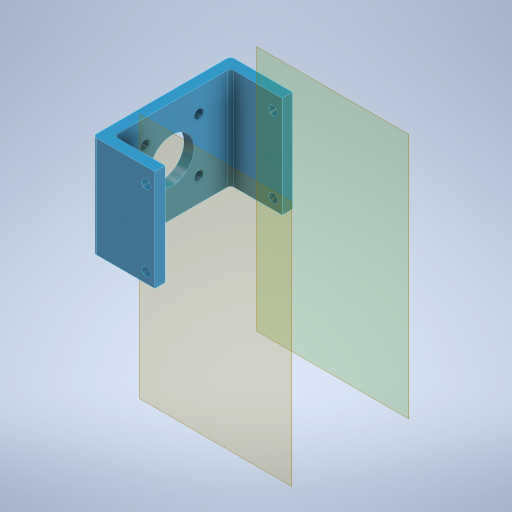
# Autodesk Inventor part: 3D_pelvis2
Saved by Autodesk Inventor 2024 (Build 280153000, 153)
## iProperties
Created: 2024-09-03
Part Number: 3D_pelvis2
Material: PMMA 플라스틱
Document SubType Name: Modeling
Designer: jmha0
Density: 1.188 g/cm^3
Appearance: 하늘색 짙음
Author: jmha0
Autodesk Inventor part; units mm, degrees
ref_plane "YZ Plane" through (0, 0, 0) normal (1, 0, 0) x (0, 1, 0)
ref_plane "XZ Plane" through (0, 0, 0) normal (0, 1, 0) x (-1, 0, 0)
ref_plane "XY Plane" through (0, 0, 0) normal (0, 0, 1) x (1, 0, 0)
ref_plane "작업 평면1" through (0, 0, -34) normal (0, 0, -1) x (-1, 0, 0)
sketch "스케치1" plane through (0, 0, -34) normal (0, 0, -1) x (-1, 0, 0)
  circle A0 centre (17.3, -18) radius 1.35 projected
  line L0 (20.1, -44.6) -> (20.1, 8.5) projected
  line L1 (14.5, -42) -> (14.5, 11.5) projected
  circle A1 centre (17.3, 4) radius 1.35 projected
  circle A2 centre (17.3, -18) radius 1.45
  circle A3 centre (17.3, 4) radius 1.45
  line L2 (14.7, -42) -> (14.7, 11.5)
  line L3 (14.7, 11.5) -> (20.1, 8.5)
  line L4 (14.7, -20.9546) -> (32.7, -20.9546)
  line L5 (32.7, -20.9546) -> (32.7, 8.5)
  line L6 (32.7, 8.5) -> (20.1, 8.5)
  line L7 (32.7, -20.9546) -> (26.7, -20.9546)
  line L8 (26.7, -20.9546) -> (26.7, 8.5)
  line L9 (26.7, 8.5) -> (32.7, 8.5)
  line L10 (32.7, 8.5) -> (32.7, -20.9546)
  line L11 (20.1, 8.5) -> (14.7, 8.5)
  point P0 (0, 0)
  dimension "d0" = 0.1
  dimension "d1" = 0.1
  dimension "d2" = 0.2
  dimension "d3" = 18
  dimension "d8" = 6
  constraints: 20 end point, 4 perpendicular, 4 point on line, 3 parallel, 2 centre point, 1 horizontal
  measures "d0" radial gap between concentric circles of A0 A2
  measures "d1" radial gap between concentric circles of A1 A3
  measures "d2" distance between parallel lines of L1 L2
  measures "d3" distance of L4.start L4.end
  measures "d8" distance of L8.end L9.end
extrude "돌출1" add sketch "스케치1" along normal blind 3 contours L4 L2 L11 L0 | L0 L6 L8 L4 | L8 L6 L5 L4 | A2 | A3
sketch "스케치2" plane through (0, 0, -34) normal (0, 0, 1) x (1, 0, 0)
  line L0 (-20.1, 8.5) -> (-14.7, 11.5) projected
  line L1 (-14.7, 8.5) -> (-14.7, -20.9546) projected
  line L2 (-20.1, -44.6) -> (-20.1, 8.5) projected
  line L3 (-32.7, 8.5) -> (-14.7, 8.5) projected
  line L4 (-32.7, -20.9546) -> (-32.7, 8.5) projected
  line L5 (-14.7, -20.9546) -> (-32.7, -20.9546) projected
  line L6 (-20.1, -20.9546) -> (-32.7, -20.9546)
  line L7 (-32.7, -20.9546) -> (-32.7, 8.5)
  line L8 (-32.7, 8.5) -> (-20.1, 8.5)
  line L9 (-20.1, 8.5) -> (-20.1, -20.9546)
  line L10 (-20.1, -20.9546) -> (-14.7, -20.9546)
  line L11 (-14.7, 11.5) -> (-20.1, 8.5)
  circle A0 centre (-17.3, -18) radius 1.45 projected
  circle A1 centre (-17.3, 4) radius 1.35 projected
  circle A2 centre (-17.3, 4) radius 1.45 projected
  circle A3 centre (-17.3, 4) radius 1.45
  circle A4 centre (-17.3, -18) radius 1.45
  point P0 (0, 0)
  constraints: 12 end point, 2 centre point, 2 coincident, 2 concentric, 2 parallel, 2 point on line, 1 collinear, 1 horizontal, 1 perpendicular
ref_plane "작업 평면2" through (0, 0, 0) normal (0, 0, 1) x (1, 0, 0)
sketch "스케치3" plane through (0, 0, 0) normal (0, 0, 1) x (1, 0, 0)
  line L0 (-32.7, 8.5) -> (-14.7, 8.5) projected
  line L1 (-32.7, -20.9546) -> (-32.7, 8.5) projected
  line L2 (-14.7, -20.9546) -> (-32.7, -20.9546) projected
  line L3 (-14.7, 8.5) -> (-14.7, -20.9546) projected
  line L4 (-20.1, -20.9546) -> (-32.7, -20.9546)
  line L5 (-32.7, -20.9546) -> (-32.7, 8.5)
  line L6 (-32.7, 8.5) -> (-20.1, 8.5)
  line L7 (-20.1, 8.5) -> (-20.1, -20.9546)
  line L8 (-32.7, -20.9546) -> (-20.1, -20.9546)
  line L9 (-20.1, -20.9546) -> (-20.1, 8.5)
  line L10 (-20.1, 8.5) -> (-32.7, 8.5)
  line L11 (-32.7, 8.5) -> (-32.7, -20.9546)
  line L12 (-20.1, -20.9546) -> (-14.7, -20.9546)
  line L13 (-14.7, 8.5) -> (-14.7, -20.9546) projected
  line L14 (-14.7, 11.5) -> (-20.1, 8.5)
  circle A0 centre (-17.3, -18) radius 1.45
  circle A1 centre (-17.3, 4) radius 1.45
  circle A2 centre (-17.3, 4) radius 1.35
  circle A3 centre (-17.3, -18) radius 1.35
  point P0 (0, 0)
  dimension "d26" = 2.7
  dimension "d27" = 2.7
  constraints: 20 end point, 4 centre point, 4 parallel, 3 horizontal, 2 coincident, 2 perpendicular, 1 point on line
  measures "d26" diameter of A2
  measures "d27" diameter of A3
extrude "돌출2" add sketch "스케치3" along normal blind 3 contours L0 L7 L2 L1 | L0 L3 L2 L7 | A0 | A1
sketch "스케치4" plane through (0, 0, -34) normal (0, 0, 1) x (1, 0, 0)
  line L0 (-14.7, -20.9546) -> (-14.7, 8.5) projected
  line L1 (-14.7, 8.5) -> (-32.7, 8.5) projected
  line L2 (-32.7, 8.5) -> (-32.7, -20.9546) projected
  line L3 (-32.7, -20.9546) -> (-14.7, -20.9546) projected
  line L4 (-32.7, 8.5) -> (-26.7, 8.5)
  line L5 (-26.7, -20.9546) -> (-32.7, -20.9546)
  line L6 (-32.7, -20.9546) -> (-32.7, 8.5)
  line L7 (-32.7, 8.5) -> (-29.7, 8.5)
  line L8 (-29.7, 8.5) -> (-29.7, -20.9546)
  line L9 (-29.7, -20.9546) -> (-32.7, -20.9546)
  line L10 (-32.7, -20.9546) -> (-32.7, 8.5)
  point P0 (0, 0)
  point P1 (-29.7, -20.9546)
  constraints: 14 end point, 3 parallel, 2 horizontal, 1 midpoint, 1 perpendicular, 1 point on line
extrude "돌출3" add sketch "스케치4" along normal up to surface (34 mm away) contours L3 L2 L1 L8
sketch "스케치5" plane through (-32.7, -20.9546, -37) normal (-1, 0, 0) x (0, 0, 1)
  line L0 (40, 29.4546) -> (0, 29.4546) projected
  line L1 (0, 0) -> (0, 29.4546) projected
  line L2 (40, 0) -> (0, 0) projected
  line L3 (40, 29.4546) -> (40, 0) projected
  line L4 (40, 0) -> (0, 0) projected
  circle A0 centre (20, 14.7273) radius 14
  arc A1 (15, 20.2502) -> (25, 20.2502) centre (20, 14.7273) ccw
  circle A2 centre (20, 14.7273) radius 1.6
  circle A3 centre (12.2218, 22.5055) radius 1.35
  circle A4 centre (27.7782, 22.5055) radius 1.35
  circle A5 centre (27.7782, 6.9491) radius 1.35
  circle A6 centre (12.2218, 6.9491) radius 1.35
  arc A7 (15.6711, 19.5089) -> (24.3289, 19.5089) centre (20, 14.7273) ccw
  circle A8 centre (20, 14.7273) radius 6.45
  point P0 (37, 20.9546)
  point P1 (24.3289, 19.5089)
  point P2 (15.6711, 19.5089)
  dimension "d20" = 3.2
  dimension "d21" = 2.7
  dimension "d22" = 2.7
  dimension "d23" = 2.7
  dimension "d24" = 2.7
  dimension "d25" = 1
  constraints: 9 centre point, 4 point on circle, 3 coincident, 1 concentric
  measures "d20" diameter of A2
  measures "d21" diameter of A3
  measures "d22" diameter of A4
  measures "d23" diameter of A5
  measures "d24" diameter of A6
  measures "d25" radial gap between concentric circles of A1 A7
extrude "돌출4" cut sketch "스케치5" against normal blind 10 contours A2 | A3 | A4 | A5 | A6 | A8 A7
fillet "모깎기1" radius 1 4 edges at (-32.7, -6.2273, 3) (-32.7, -6.2273, -37) (-29.7, -6.2273, -34) (-29.7, -6.2273, 0)
